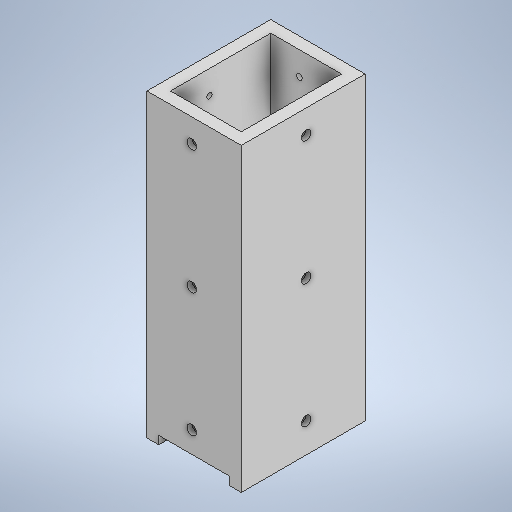
# Autodesk Inventor part: TS_V1_Fallmagazin_Wandung_int
Saved by Autodesk Inventor 2025.2 (Build 292293000, 293)
## iProperties
Created: 2025-06-10
Part Number: TS_V1_Fallmagazin_Wandung_int
Material: Generisch
Document SubType Name: Modeling
Designer: tino
Density: 1 g/cm^3
Appearance: Vorgabe
Author: tino
Autodesk Inventor part; units mm, degrees
ref_plane "YZ Plane" through (0, 0, 0) normal (1, 0, 0) x (0, 1, 0)
ref_plane "XZ Plane" through (0, 0, 0) normal (0, 1, 0) x (-1, 0, 0)
ref_plane "XY Plane" through (0, 0, 0) normal (0, 0, 1) x (1, 0, 0)
sketch "Skizze1" plane through (0, 0, 0) normal (0, 0, 1) x (1, 0, 0)
  spline S0 degree 3 poles (4.1682, 35.1897) (1.1905, 36.4598) (-2.2497, 35.1642) (-6.2549, 34.1582) (-11.7361, 32.1479) (-17.2675, 27.437) (-17.3979, 22.2805) (-19.1794, 11.8373) (-24.2043, -4.2198) (-21.9122, -21.3618) (-15.7263, -32.1361) (-8.9601, -34.8731) (-7.7344, -35.2068) knots 0 0 0 0 0.05535 0.076528 0.211782 0.295547 0.382964 0.432922 0.754884 0.81234 0.967238 1 1 1 1
  spline S1 degree 3 poles (-7.7344, -35.2068) (-2.4391, -36.6482) (4.9342, -35.145) (14.3889, -31.3641) (20.2206, -28.2766) (23.0847, -23.1792) (23.281, -18.9959) (17.3062, -16.4997) (13.7398, -19.2937) (6.9074, -22.9332) (-1.1986, -27.1621) (-10.3055, -22.9326) (-14.0352, -10.4002) (-9.4599, -0.926) (-6.8333, 0.3153) (-5.9182, 2.0588) (-5.9367, 4.1791) (-8.2887, 5.2306) (-8.3641, 10.4373) (-1.0106, 14.1251) (4.0821, 20.0507) (3.0635, 26.3026) (2.9493, 28.6136) (3.7888, 29.834) (5.5778, 31.0924) (6.6132, 32.7745) (5.2458, 34.7086) (4.2657, 35.1481) (4.1682, 35.1897) knots 0 0 0 0 0.14153 0.17035 0.245987 0.25892 0.290227 0.326265 0.372233 0.38898 0.482096 0.508256 0.624416 0.647418 0.715274 0.72607 0.746892 0.801722 0.811885 0.848514 0.916356 0.943374 0.948219 0.962959 0.96651 0.98188 0.998188 1 1 1 1
  arc A0 (-7.9107, 24.207) -> (-7.9109, 20.407) centre (-6.0635, 22.307) ccw
  line L0 (-7.9107, 24.207) -> (-4.2161, 24.2069)
  arc A1 (-4.2163, 20.4069) -> (-4.2161, 24.2069) centre (-6.0635, 22.307) ccw
  line L1 (-4.2163, 20.4069) -> (-7.9109, 20.407)
  spline S2 degree 3 poles (4.1682, 35.1897) (1.1905, 36.4598) (-2.2497, 35.1642) (-6.255, 34.1582) (-11.7361, 32.1479) (-17.2675, 27.437) (-17.3979, 22.2805) (-19.1794, 11.8373) (-24.2043, -4.2198) (-21.9122, -21.3619) (-15.7263, -32.1361) (-8.9601, -34.8731) (-7.7344, -35.2068) knots 0 0 0 0 0.05535 0.076528 0.211782 0.295547 0.382964 0.432922 0.754884 0.81234 0.967238 1 1 1 1
  spline S3 degree 3 poles (-7.7344, -35.2068) (-2.4391, -36.6482) (4.9342, -35.145) (14.3889, -31.3641) (20.2206, -28.2766) (23.0847, -23.1792) (23.281, -18.9959) (17.3062, -16.4997) (13.7398, -19.2937) (6.9074, -22.9332) (-1.1986, -27.1621) (-10.3055, -22.9326) (-14.0352, -10.4002) (-9.4599, -0.926) (-6.8333, 0.3153) (-5.9182, 2.0588) (-5.9367, 4.1791) (-8.2887, 5.2306) (-8.3641, 10.4373) (-1.0106, 14.1251) (4.0821, 20.0507) (3.0635, 26.3026) (2.9493, 28.6136) (3.7888, 29.834) (5.5778, 31.0924) (6.6132, 32.7745) (5.2458, 34.7086) (4.2657, 35.1481) (4.1682, 35.1897) knots 0 0 0 0 0.14153 0.17035 0.245987 0.25892 0.290227 0.326265 0.372233 0.38898 0.482096 0.508256 0.624416 0.647418 0.715274 0.72607 0.746892 0.801722 0.811885 0.848514 0.916356 0.943374 0.948219 0.962959 0.96651 0.98188 0.998188 1 1 1 1
  line L2 (-4.2163, 20.4069) -> (-7.9109, 20.407)
  arc A2 (-4.2163, 20.4069) -> (-4.2161, 24.2069) centre (-6.0635, 22.307) ccw
  line L3 (-7.9107, 24.207) -> (-4.2161, 24.2069)
  arc A3 (-7.9107, 24.207) -> (-7.9109, 20.407) centre (-6.0635, 22.307) ccw
  line L4 (-22.9949, 35.8296) -> (22.9949, 35.8296) construction
  line L5 (22.9949, 35.8296) -> (22.9949, -35.8296) construction
  line L6 (22.9949, -35.8296) -> (-22.9949, -35.8296) construction
  line L7 (-22.9949, -35.8296) -> (-22.9949, 35.8296) construction
  line L8 (-22.9949, 35.8296) -> (22.9949, -35.8296) construction
  line L9 (-22.9949, -35.8296) -> (22.9949, 35.8296) construction
  point P0 (0, 0)
  point P1 (-38.8867, -20.8658)
  point P2 (0, 0)
  constraints: 20 end point, 8 point on circle, 4 centre point, 3 horizontal, 3 perpendicular, 2 vertical, 1 midpoint, 8 other
sketch "Skizze2" plane through (0, 0, 0) normal (0, 0, 1) x (1, 0, 0)
  line L0 (-30, 42.5) -> (30, 42.5)
  line L1 (30, 42.5) -> (30, -42.5)
  line L2 (30, -42.5) -> (-30, -42.5)
  line L3 (-30, -42.5) -> (-30, 42.5)
  line L4 (-30, 42.5) -> (30, -42.5) construction
  line L5 (30, 42.5) -> (-30, -42.5) construction
  arc A0 (-7.9107, 24.207) -> (-7.9109, 20.407) centre (-6.0635, 22.307) ccw
  arc A1 (-7.9107, 24.207) -> (-7.9109, 20.407) centre (-6.0635, 22.307) ccw
  line L6 (-7.9107, 24.207) -> (-4.2161, 24.2069)
  line L7 (-7.9107, 24.207) -> (-4.2161, 24.2069)
  line L8 (-4.2163, 20.4069) -> (-7.9109, 20.407)
  line L9 (-4.2163, 20.4069) -> (-7.9109, 20.407)
  arc A2 (-4.2163, 20.4069) -> (-4.2161, 24.2069) centre (-6.0635, 22.307) ccw
  arc A3 (-4.2163, 20.4069) -> (-4.2161, 24.2069) centre (-6.0635, 22.307) ccw
  line L10 (-22.9949, 35.8296) -> (22.9949, 35.8296) construction
  line L11 (-22.9949, -35.8296) -> (-22.9949, 35.8296) construction
  spline S0 degree 3 poles (4.1682, 35.1897) (1.1905, 36.4598) (-2.2497, 35.1642) (-6.255, 34.1582) (-11.7361, 32.1479) (-17.2675, 27.437) (-17.3979, 22.2805) (-19.1794, 11.8373) (-24.2043, -4.2198) (-21.9122, -21.3619) (-15.7263, -32.1361) (-8.9601, -34.8731) (-7.7344, -35.2068) knots 0 0 0 0 0.05535 0.076528 0.211782 0.295547 0.382964 0.432922 0.754884 0.81234 0.967238 1 1 1 1
  spline S1 degree 3 poles (4.1682, 35.1897) (1.1905, 36.4598) (-2.2497, 35.1642) (-6.2549, 34.1582) (-11.7361, 32.1479) (-17.2675, 27.437) (-17.3979, 22.2805) (-19.1794, 11.8373) (-24.2043, -4.2198) (-21.9122, -21.3618) (-15.7263, -32.1361) (-8.9601, -34.8731) (-7.7344, -35.2068) knots 0 0 0 0 0.05535 0.076528 0.211782 0.295547 0.382964 0.432922 0.754884 0.81234 0.967238 1 1 1 1
  line L12 (-22.9949, 35.8296) -> (22.9949, -35.8296) construction
  line L13 (-22.9949, -35.8296) -> (22.9949, 35.8296) construction
  line L14 (22.9949, -35.8296) -> (-22.9949, -35.8296) construction
  spline S2 degree 3 poles (-7.7344, -35.2068) (-2.4391, -36.6482) (4.9342, -35.145) (14.3889, -31.3641) (20.2206, -28.2766) (23.0847, -23.1792) (23.281, -18.9959) (17.3062, -16.4997) (13.7398, -19.2937) (6.9074, -22.9332) (-1.1986, -27.1621) (-10.3055, -22.9326) (-14.0352, -10.4002) (-9.4599, -0.926) (-6.8333, 0.3153) (-5.9182, 2.0588) (-5.9367, 4.1791) (-8.2887, 5.2306) (-8.3641, 10.4373) (-1.0106, 14.1251) (4.0821, 20.0507) (3.0635, 26.3026) (2.9493, 28.6136) (3.7888, 29.834) (5.5778, 31.0924) (6.6132, 32.7745) (5.2458, 34.7086) (4.2657, 35.1481) (4.1682, 35.1897) knots 0 0 0 0 0.14153 0.17035 0.245987 0.25892 0.290227 0.326265 0.372233 0.38898 0.482096 0.508256 0.624416 0.647418 0.715274 0.72607 0.746892 0.801722 0.811885 0.848514 0.916356 0.943374 0.948219 0.962959 0.96651 0.98188 0.998188 1 1 1 1
  spline S3 degree 3 poles (-7.7344, -35.2068) (-2.4391, -36.6482) (4.9342, -35.145) (14.3889, -31.3641) (20.2206, -28.2766) (23.0847, -23.1792) (23.281, -18.9959) (17.3062, -16.4997) (13.7398, -19.2937) (6.9074, -22.9332) (-1.1986, -27.1621) (-10.3055, -22.9326) (-14.0352, -10.4002) (-9.4599, -0.926) (-6.8333, 0.3153) (-5.9182, 2.0588) (-5.9367, 4.1791) (-8.2887, 5.2306) (-8.3641, 10.4373) (-1.0106, 14.1251) (4.0821, 20.0507) (3.0635, 26.3026) (2.9493, 28.6136) (3.7888, 29.834) (5.5778, 31.0924) (6.6132, 32.7745) (5.2458, 34.7086) (4.2657, 35.1481) (4.1682, 35.1897) knots 0 0 0 0 0.14153 0.17035 0.245987 0.25892 0.290227 0.326265 0.372233 0.38898 0.482096 0.508256 0.624416 0.647418 0.715274 0.72607 0.746892 0.801722 0.811885 0.848514 0.916356 0.943374 0.948219 0.962959 0.96651 0.98188 0.998188 1 1 1 1
  line L15 (22.9949, 35.8296) -> (22.9949, -35.8296) construction
  line L16 (-40, 52.5) -> (40, 52.5)
  line L17 (40, 52.5) -> (40, -52.5)
  line L18 (40, -52.5) -> (-40, -52.5)
  line L19 (-40, -52.5) -> (-40, 52.5)
  line L20 (-40, 52.5) -> (40, -52.5) construction
  line L21 (40, 52.5) -> (-40, -52.5) construction
  point P0 (0, 0)
  point P1 (0, 0)
  point P2 (-38.8867, -20.8658)
  point P3 (0, 0)
  dimension "d0" = 45.9898
  dimension "d1" = 71.6591
  dimension "d2" = 60
  dimension "d3" = 85
  dimension "d4" = 80
  dimension "d5" = 105
  constraints: 24 end point, 4 midpoint, 4 parallel, 2 horizontal, 2 perpendicular
  measures "d0" distance between parallel lines of L15 L11
  measures "d1" distance of L11.start L10.start
  measures "d2" distance of L0.start L0.end
  measures "d3" distance of L2.end L0.start
  measures "d4" distance of L17.end L18.end
  measures "d5" distance of L16.end L17.end
extrude "Extrusion1" add sketch "Skizze2" along normal blind 255 contours L16 L17 L18 L19
sketch "Skizze3" plane through (-40, -52.5, 0) normal (0, -1, 0) x (1, 0, 0)
  line L0 (80, 0) -> (0, 0) projected
  line L1 (10, 0) -> (70, 0)
  line L2 (70, 0) -> (70, 5)
  line L3 (70, 5) -> (10, 5)
  line L4 (10, 5) -> (10, 0)
  line L5 (40, 5) -> (40, 0) construction
  point P0 (40, 0)
  point P1 (70, 0)
  dimension "d8" = 60
  dimension "d9" = 5
  constraints: 10 end point, 3 midpoint, 2 parallel, 2 point on line, 1 horizontal, 1 perpendicular
  measures "d8" distance of L3.end L2.end
  measures "d9" distance of L1.end L2.end
extrude "Extrusion2" cut sketch "Skizze3" against normal blind 105
sketch "Skizze4" plane through (0, 0, 0) normal (0, 0, -1) x (-1, 0, 0)
  point P0 (0, 0)
  point P1 (35, -47.5)
  dimension "d12" = 47.5
  dimension "d13" = 35
  measures "d12" vertical distance of point (35, -47.5) point (0, 0)
  measures "d13" horizontal distance of point (0, 0) point (35, -47.5)
hole "Bohrung1" at (-35, -47.5, 0) direction (0, 0, 1) diameter 3.242 depth 11.8 tip angle 118 thread size "M4x0.7" class "6H" standard "ISO Metric profile"
chamfer "Fasen1" distance 1 angle 45 1 edges at (-35, -49.121, 0)
pattern_linear "Rechteckige Anordnung1" count 2 spacing 70 along (1, 0, 0) count 3 spacing 47.5 along (0, 1, 0) of "Bohrung1", "Fasen1"
sketch "Skizze5" plane through (40, -52.5, 0) normal (1, 0, 0) x (0, 0, -1)
  line L0 (0, 105) -> (-255, 105) projected
  line L1 (-255, 0) -> (-255, 105) projected
  line L2 (0, 0) -> (0, 105) projected
  line L3 (0, 0) -> (-255, 0) projected
  line L4 (-5, 95) -> (-255, 95) projected
  point P0 (0, 52.5)
  point P1 (-235, 55.1)
  point P2 (-130, 55.1)
  point P3 (-25, 55.1)
  point P4 (-255, 52.5)
  dimension "d31" = 20
  dimension "d32" = 125
  dimension "d33" = 25
  dimension "d42" = 39.9
  constraints: 2 horizontal alignment, 1 midpoint
  measures "d31" horizontal distance of point (-235, 55.1) point (-255, 52.5)
  measures "d32" distance from line of point (-130, 55.1) L1
  measures "d33" distance from line of L2 point (-25, 55.1)
  measures "d42" distance from line of L4 point (-235, 55.1)
hole "Bohrung2" at (40, 2.6, 235) at (40, 2.6, 130) at (40, 2.6, 25) direction (-1, 0, 0) diameter 4.5 depth 10 tip angle 118 counterbore diameter 8 counterbore depth 4.4
sketch "Skizze6" plane through (-40, 52.5, 0) normal (0, 1, 0) x (1, 0, 0)
  line L0 (80, -126) -> (80, -134) projected
  line L1 (80, -231) -> (80, -239) projected
  line L2 (80, -21) -> (80, -29) projected
  line L3 (10, -5) -> (10, -255) projected
  point P0 (40, 0)
  point P1 (80, -235)
  point P2 (34.4, -235)
  point P3 (80, -130)
  point P4 (34.4, -130)
  point P5 (80, -25)
  point P6 (34.4, -25)
  dimension "d43" = 24.4
  constraints: 3 horizontal alignment, 3 midpoint, 2 vertical alignment
  measures "d43" distance from line of L3 point (34.4, -235)
hole "Bohrung3" at (-5.6, 52.5, 235) at (-5.6, 52.5, 130) at (-5.6, 52.5, 25) direction (0, -1, 0) diameter 4.5 depth 10 tip angle 118 counterbore diameter 8 counterbore depth 4.4
sketch "Skizze7" plane through (-40, -52.5, 0) normal (-1, 0, 0) x (0, 0, 1)
  line L0 (231, 105) -> (239, 105) projected
  line L1 (126, 105) -> (134, 105) projected
  line L2 (21, 105) -> (29, 105) projected
  line L3 (5, 95) -> (255, 95) projected
  line L4 (5, 10) -> (255, 10) projected
  point P0 (0, 52.5)
  point P1 (235, 105)
  point P2 (235, 43)
  point P3 (130, 43)
  point P4 (25, 43)
  point P5 (130, 105)
  point P6 (25, 105)
  dimension "d67" = 33
  constraints: 3 midpoint, 3 vertical alignment, 2 horizontal alignment
  measures "d67" distance from line of L4 point (235, 43)
hole "Bohrung4" at (-40, -9.5, 235) at (-40, -9.5, 130) at (-40, -9.5, 25) direction (1, 0, 0) diameter 4.5 depth 10 tip angle 118 counterbore diameter 8 counterbore depth 4.4
sketch "Skizze8" plane through (30, -52.5, 0) normal (0, -1, 0) x (1, 0, 0)
  circle A0 centre (-35.6, 235) radius 2.25 projected
  circle A1 centre (-35.6, 130) radius 2.25 projected
  circle A2 centre (-35.6, 25) radius 2.25 projected
  circle A3 centre (-35.6, 130) radius 4 projected
  line L0 (-60, 5) -> (-60, 255) projected
  line L1 (-70, 231) -> (-70, 239) projected
  point P0 (-30, 0)
  point P1 (-32, 235)
  point P2 (-32, 130)
  point P3 (-32, 25)
  point P4 (-34.5692, 20)
  point P5 (-36.6308, 20)
  point P6 (-70, 235)
  dimension "d59" = 28
  constraints: 4 horizontal alignment, 3 coincident, 2 vertical alignment, 1 midpoint, 1 other
  measures "d59" distance from line of L0 point (-32, 235)
hole "Bohrung5" at (-2, -52.5, 25) at (-2, -52.5, 130) at (-2, -52.5, 235) direction (0, 1, 0) diameter 4.5 depth 10 tip angle 118 counterbore diameter 8 counterbore depth 4.4
chamfer "Fasen2" distance 2 angle 45 2 edges at (0, -52.5, 5) (0, 52.5, 5)
sketch "Skizze9" plane through (0, 0, 0) normal (0, 0, -1) x (-1, 0, 0)
  circle A0 centre (35, -47.5) radius 1.621 projected
  circle A1 centre (35, 0) radius 1.621 projected
  circle A2 centre (-35, 0) radius 1.621 projected
  point P0 (0, 0)
  point P1 (35, 23.75)
  point P2 (-35, -23.75)
  dimension "d71" = 47.5
  dimension "d81" = 23.75
  dimension "d82" = 23.75
  constraints: 2 vertical alignment
  measures "d71" distance of A1.centre A0.centre
  measures "d81" distance of A2.centre point (-35, -23.75)
  measures "d82" distance of point (35, 23.75) A1.centre
hole "Bohrung6" at (-35, 23.75, 0) at (35, -23.75, 0) direction (0, 0, 1) diameter 4 depth 5.5 countersink diameter 5 countersink angle 90
equation "\"d2\" = Breite_innen"
equation "\"d3\" = Laenge_innen"
equation "\"d4\" = Breite_aussen"
equation "\"d5\" = Laenge_aussen"
equation "\"d6\" = Hoehe_Magazin"
equation "\"d8\" = Breite_innen"
equation "\"d9\" = Ausschubhoehe"
equation "\"d10\" = Laenge_aussen"
equation "\"d12\" = -0.5 * Wanddicke + 0.5 * Laenge_aussen"
equation "\"d13\" = -0.5 * Wanddicke + 0.5 * Breite_aussen"
equation "\"d26\" = Breite_aussen - Wanddicke"
equation "\"d29\" = -0.5 * Wanddicke + 0.5 * Laenge_aussen"
equation "\"d31\" = Abstand_Rand"
equation "\"d32\" = -0.5 * Ausschubhoehe + 0.5 * Hoehe_Magazin"
equation "\"d33\" = d31 + Absatz"
equation "\"d49\" = Wanddicke"
equation "\"d57\" = Wanddicke"
equation "\"d65\" = Wanddicke"
equation "\"d81\" = d72"
equation "\"d82\" = d81"
equation "\"Breite_innen\" = 60"
equation "\"Laenge_innen\" = 85"
equation "\"Breite_aussen\" = Breite_innen + 2 * Wanddicke"
equation "\"Laenge_aussen\" = Laenge_innen + 2 * Wanddicke"
equation "\"Wanddicke\" = 10"
equation "\"Ausschubhoehe\" = Absatz"
equation "\"Absatz\" = 5"
equation "\"Abstand_Rand\" = 20"
equation "\"d72\" = 0.5 * d71"
equation "\"Hoehe_Magazin\" = 255"
